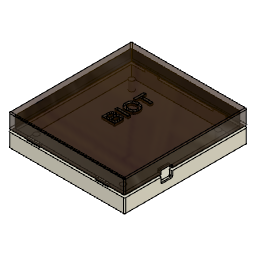
BIOT-caja (Autodesk Fusion 360 design; units mm, degrees)
Autodesk Fusion 360 part; units mm, degrees
box "BoxPrimitive1" add length 107.41 width 101.06 height 21 placed x (0, 1, 0) y (-1, 0, 0) z (0, 0, 1) at (103.6056, 2.803, 0) makes body 1
shell "Shell1" thickness 3 outward yes removed faces 0 bodies 1
sketch "Sketch2" plane through (106.6056, 0, 0) normal (1, 0, 0) x (0, 1, 0)
  line L0 (-0.197, 24) -> (-0.197, -3)
  line L1 (-0.197, -3) -> (113.213, -3)
  line L2 (113.213, -3) -> (113.213, 24)
  line L3 (113.213, 24) -> (-0.197, 24)
  line L4 (43.62, 8.68) -> (34, 8.68)
  line L5 (34, 8.68) -> (34, 16)
  line L6 (34, 16) -> (43.62, 16)
  line L7 (43.62, 16) -> (43.62, 8.68)
move_body "Move1" bodies 1 to x (1, 0, 0) y (0, 1, 0) z (0, 0, 1) at (0, 0, 3)
extrude "Extrude1" cut sketch "Sketch2" against normal blind 10 contours L4 L5 L6 L7 bodies 1
fillet "Fillet1" radius 0.6 4 faces at (105.6056, 40.4133, 8.68) (105.6056, 34, 11.12) (105.6056, 43.62, 13.56) (105.6056, 37.2067, 16) on bodies 1
fillet "Fillet2" radius 1 31 faces at (35.2322, 37.6063, 27) (106.6056, 90.2153, 14.1333) (106.6049, 33.7522, 8.4716) (105.4056, 34.4585, 8.6969) (103.6063, 34.0143, 8.2655) (103.6056, 88.2153, 14.1333) (103.9056, 37.4067, 8.5996) (103.6063, 43.6995, 8.3258) (105.4056, 43.1615, 8.6969) (105.4056, 40.2133, 8.68) (106.3056, 40.2133, 8.5996) (106.6049, 43.6995, 8.3258) (106.2805, 43.6867, 13.36) (106.6049, 43.6057, 16.4145) (105.4056, 43.243, 15.957) (103.6063, 43.6057, 16.4145) (103.9306, 43.6867, 11.32) (105.4056, 43.62, 13.36) (103.9056, 40.2133, 16.0804) (103.6063, 33.5588, 15.9368) (104.8056, 34.4585, 15.9831) (105.4056, 37.4067, 16) (106.3056, 37.4067, 16.0804) (106.6049, 34.0143, 16.4145) (106.2805, 33.9333, 11.32) (105.4056, 34, 11.32) (103.9306, 33.9333, 13.36) (35.2322, 113.213, 9) (-0.4544, 37.6063, 9) (35.2322, -0.197, 9) (35.2322, 37.6063, 0) on bodies 1
ref_plane "WorkPlane1" through (53.0756, 56.508, 13.5) normal (0, 0, 1) x (0, 1, 0)
split "Split1" by plane through (53.0756, 56.508, 13.5) normal (0, 0, 1) bodies 1 makes body 2 at (70.5856, 75.0763, 27)
copy_body "Body->Comp1" bodies 1 removing the originals makes body 3 in component "Component"
copy_body "Body->Comp2" bodies 2 removing the originals makes body 4 in component "Component'"
sketch "Sketch3" plane through (0, 0, 3) normal (0, 0, 1) x (-1, 0, 0)
  line L0 (-102.6056, -2.803) -> (-102.6056, -110.213)
  line L1 (-102.6056, -110.213) -> (-2.5456, -110.213)
  line L2 (-2.5456, -110.213) -> (-2.5456, -2.803)
  line L3 (-2.5456, -2.803) -> (-102.6056, -2.803)
  circle A0 centre (-12.5, -12.5) radius 2.5
  circle A1 centre (-12.5, -100.5) radius 2.5
  circle A2 centre (-92.5, -12.5) radius 2.5
  circle A3 centre (-93, -100) radius 2.5
sketch "Sketch4" plane through (0, 0, 3) normal (0, 0, 1) x (1, 0, 0)
sketch "Sketch5" plane through (0, 0, 3) normal (0, 0, 1) x (-1, 0, 0)
extrude "Extrude1'" add sketch "Sketch3" along normal blind 8.5 contours A0 | A1 | A2 | A3 bodies 3 in component "Component"
sketch "Sketch6" plane through (0, 0, 13.5) normal (0, 0, 1) x (-1, 0, 0)
  arc A0 (0.4544, -0.803) -> (-0.5456, 0.197) centre (-0.5456, -0.803) ccw
  line L0 (-0.5456, 0.197) -> (-105.6056, 0.197)
  arc A1 (-105.6056, 0.197) -> (-106.6056, -0.803) centre (-105.6056, -0.803) ccw
  line L1 (-106.6056, -0.803) -> (-106.6056, -33.4)
  arc A2 (-106.6056, -33.4) -> (-106.0056, -34) centre (-106.0056, -33.4) ccw
  line L2 (-106.0056, -34) -> (-104.2056, -34)
  arc A3 (-104.2056, -34) -> (-103.6056, -33.4) centre (-104.2056, -33.4) ccw
  line L3 (-103.6056, -33.4) -> (-103.6056, -3.803)
  arc A4 (-102.6056, -2.803) -> (-103.6056, -3.803) centre (-102.6056, -3.803) ccw
  line L4 (-102.6056, -2.803) -> (-2.5456, -2.803)
  line L5 (-2.5456, -2.803) -> (-2.5456, -110.213)
  line L6 (-2.5456, -110.213) -> (-102.6056, -110.213)
  arc A5 (-103.6056, -109.213) -> (-102.6056, -110.213) centre (-102.6056, -109.213) ccw
  line L7 (-103.6056, -109.213) -> (-103.6056, -44.22)
  arc A6 (-103.6056, -44.22) -> (-104.2056, -43.62) centre (-104.2056, -44.22) ccw
  line L8 (-104.2056, -43.62) -> (-106.0056, -43.62)
  arc A7 (-106.0056, -43.62) -> (-106.6056, -44.22) centre (-106.0056, -44.22) ccw
  line L9 (-106.6056, -44.22) -> (-106.6056, -112.213)
  arc A8 (-106.6056, -112.213) -> (-105.6056, -113.213) centre (-105.6056, -112.213) ccw
  line L10 (-105.6056, -113.213) -> (-0.5456, -113.213)
  arc A9 (-0.5456, -113.213) -> (0.4544, -112.213) centre (-0.5456, -112.213) ccw
  line L11 (0.4544, -112.213) -> (0.4544, -0.803)
  line L12 (-14.9946, -2.803) -> (-26.9946, -2.803)
  line L13 (-26.9946, -2.803) -> (-26.9946, -1.303)
  line L14 (-26.9946, -1.303) -> (-14.9946, -1.303)
  line L15 (-14.9946, -1.303) -> (-14.9946, -2.803)
  line L16 (-90.0122, -2.803) -> (-78.0122, -2.803)
  line L17 (-78.0122, -2.803) -> (-78.0122, -1.303)
  line L18 (-78.0122, -1.303) -> (-90.0122, -1.303)
  line L19 (-90.0122, -1.303) -> (-90.0122, -2.803)
  line L20 (-89.9351, -110.213) -> (-77.9351, -110.213)
  line L21 (-77.9351, -110.213) -> (-77.9351, -111.713)
  line L22 (-77.9351, -111.713) -> (-89.9351, -111.713)
  line L23 (-89.9351, -111.713) -> (-89.9351, -110.213)
  line L24 (-14.9393, -110.213) -> (-26.9393, -110.213)
  line L25 (-26.9393, -110.213) -> (-26.9393, -111.713)
  line L26 (-26.9393, -111.713) -> (-14.9393, -111.713)
  line L27 (-14.9393, -111.713) -> (-14.9393, -110.213)
  constraint horizontal L12
  constraint vertical L13
  constraint horizontal L14
  constraint vertical L15
  constraint coincident L4 L12.start
  constraint horizontal L16
  constraint vertical L17
  constraint horizontal L18
  constraint vertical L19
  constraint coincident L4 L16.start
  constraint horizontal L20
  constraint vertical L21
  constraint horizontal L22
  constraint vertical L23
  constraint coincident L6 L20.start
  constraint horizontal L24
  constraint vertical L25
  constraint horizontal L26
  constraint vertical L27
  constraint coincident L6 L24.start
extrude "Extrude2" add sketch "Sketch6" along normal blind 2.5 contours L4 L16 L17 L18 L19 | L6 L20 L21 L22 L23 | L4 L12 L13 L14 L15 | L6 L24 L25 L26 L27 bodies 3 in component "Component"
sketch "Sketch7" plane through (0, 0, 29.3) normal (0, 0, 1) x (-1, 0, 0)
  line L0 (-105.6056, -112.213) -> (-0.5456, -112.213)
  line L1 (-0.5456, -112.213) -> (-0.5456, -0.803)
  line L2 (-0.5456, -0.803) -> (-105.6056, -0.803)
  line L3 (-105.6056, -0.803) -> (-105.6056, -112.213)
  line L4 (-61.1555, -38.7374) -> (-61.6557, -77.6376) construction
  line L5 (-61.6557, -77.6376) -> (-46.7309, -77.8295) construction
  line L6 (-46.7309, -77.8295) -> (-46.2307, -38.9293) construction
  line L7 (-46.2307, -38.9293) -> (-61.1555, -38.7374) construction
  text T0 "BIOT\n" font "Arial" height 12 bold align centre top in box 38.9034 x 14.926 at (-61.1555, -38.7374) x (-0.012857, -0.999917) y (0.999917, -0.012857) spacing 1 kerned
extrude "Extrude1''" cut sketch "Sketch7" against normal blind 2 text T0 sketch seen with x (1, 0, 0) y (0, 1, 0) z (0, 0, 1) at (0, 0, -2.3) bodies 4 in component "Component'"
component "Component" placed x (1, 0, 0) y (0, 1, 0) z (0, 0, 1) at (0, 0, 0)
component "Component'" placed x (1, 0, 0) y (0, 1, 0) z (0, 0, 1) at (0, 0, 2.3)
